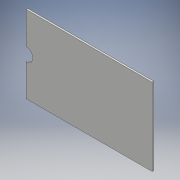
# Autodesk Inventor part: COVER_revised
Saved by Autodesk Inventor 2019 (Build 230136000, 136)
## iProperties
Part Number: COVER_revised
Material: 一般
Document SubType Name: Modeling
Designer: KazutoDell
Density: 1 g/cm^3
Appearance: 既定
Author: KazutoDell
Autodesk Inventor part; units mm, degrees
ref_plane "YZ Plane" through (0, 0, 0) normal (1, 0, 0) x (0, 1, 0)
ref_plane "XZ Plane" through (0, 0, 0) normal (0, 1, 0) x (-1, 0, 0)
ref_plane "XY Plane" through (0, 0, 0) normal (0, 0, 1) x (1, 0, 0)
sketch "スケッチ1" plane through (0, 0, 0) normal (0, 1, 0) x (-1, 0, 0)
  line L0 (0, 0) -> (-114, 0)
  line L1 (-114, 0) -> (-114, -70)
  line L2 (-114, -70) -> (0, -70)
  line L3 (0, -70) -> (0, 0)
  dimension "d0" = 114
  dimension "d1" = 70
  constraints: 8 end point, 2 parallel, 1 horizontal, 1 perpendicular
  measures "d0" distance of L2.end L1.end
  measures "d1" distance of L1.end L0.end
extrude "押し出し1" add sketch "スケッチ1" along normal blind 1.5
sketch "スケッチ2" plane through (0, 1.5, 0) normal (0, 1, 0) x (1, 0, 0)
  line L0 (0, 70) -> (0, 0) projected
  circle A0 centre (0, 35) radius 6
  dimension "d4" = 12
  constraints: 1 centre point, 1 midpoint
  measures "d4" diameter of A0
extrude "押し出し2" cut sketch "スケッチ2" against normal blind 3
